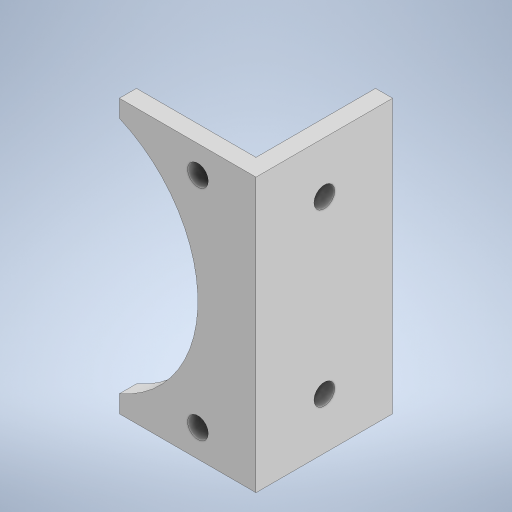
# Autodesk Inventor part: Frame Bracket
Saved by Autodesk Inventor 2023 (Build 270158000, 158)
## iProperties
Created: 2022-10-26
Part Number: Frame Bracket
Material: Generic
Document SubType Name: Modeling
Designer: tommy
Density: 1 g/cm^3
Appearance: Default
Author: tommy
Autodesk Inventor part; units mm, degrees
ref_plane "YZ Plane" through (0, 0, 0) normal (1, 0, 0) x (0, 1, 0)
ref_plane "XZ Plane" through (0, 0, 0) normal (0, 1, 0) x (-1, 0, 0)
ref_plane "XY Plane" through (0, 0, 0) normal (0, 0, 1) x (1, 0, 0)
sketch "Sketch1" plane through (0, 0, 0) normal (0, 1, 0) x (-1, 0, 0)
  line L0 (0, 0) -> (0, -25.4)
  line L1 (0, -25.4) -> (3.175, -25.4)
  line L2 (3.175, -25.4) -> (3.175, -3.175)
  line L3 (3.175, -3.175) -> (25.4, -3.175)
  line L4 (25.4, -3.175) -> (25.4, 0)
  line L5 (25.4, 0) -> (0, 0)
  dimension "d0" = 25.4
  dimension "d1" = 3.175
  dimension "d2" = 22.225
  dimension "d3" = 22.225
  constraints: 12 end point, 5 perpendicular, 1 vertical
  measures "d0" distance of L0.start L0.end
  measures "d1" distance of L0.end L1.end
  measures "d2" distance of L1.end L2.end
  measures "d3" distance of L2.end L3.end
extrude "Extrusion1" add sketch "Sketch1" along normal blind 50.8
sketch "Sketch2" plane through (-25.4, 0, 0) normal (0, 0, 1) x (1, 0, 0)
  line L0 (22.225, 0) -> (22.225, 50.8) projected
  line L1 (22.225, 0) -> (0, 0) projected
  line L2 (22.225, 50.8) -> (0, 50.8) projected
  circle A0 centre (14.605, 45.72) radius 1.9304
  circle A1 centre (14.605, 5.08) radius 1.9304
  circle A2 centre (-9.525, 25.4) radius 24.13
  line L3 (25.4, 0) -> (22.225, 0) projected
  dimension "d9" = 3.8608
  dimension "d10" = 3.8608
  constraints: 3 centre point
  measures "d9" diameter of A0
  measures "d10" diameter of A1
extrude "Extrusion2" cut sketch "Sketch2" against normal blind 63.5
sketch "Sketch3" plane through (0, 0, 0) normal (1, 0, 0) x (0, 0, -1)
  line L0 (25.4, 0) -> (25.4, 50.8) projected
  line L1 (0, 3.2295) -> (0, 47.5705) projected
  line L2 (0, 50.8) -> (25.4, 50.8) projected
  line L3 (25.4, 0) -> (3.175, 0) projected
  circle A0 centre (12.7, 9.525) radius 1.9304
  circle A1 centre (12.7, 41.275) radius 1.9304
  point P0 (0, 0)
  point P1 (12.7, 50.8)
  point P2 (14.2875, 0)
  dimension "d29" = 9.525
  dimension "d30" = 12.7
  dimension "d31" = 9.525
  dimension "d32" = 12.7
  dimension "d33" = 3.8608
  dimension "d34" = 3.8608
  constraints: 2 centre point, 2 midpoint
  measures "d29" distance of point (12.7, 50.8) A1.centre
  measures "d30" distance from line of L1 A1.centre
  measures "d31" vertical distance of point (14.287, 0) A0.centre
  measures "d32" distance from line of L1 A0.centre
  measures "d33" diameter of A0
  measures "d34" diameter of A1
extrude "Extrusion3" cut sketch "Sketch3" against normal blind 63.5
body "Solid1"
